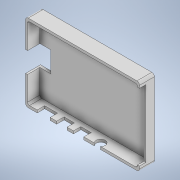
# Autodesk Inventor part: Pi 4 Case - Back Panel
Saved by Autodesk Inventor 2020 (Build 240168000, 168)
## iProperties
Created: 2021-01-01
Part Number: Pi 4 Case - Back Panel
Material: Generic
Document SubType Name: Modeling
Designer: frost
Density: 1 g/cm^3
Appearance: Default
Author: frost
Autodesk Inventor part; units mm, degrees
ref_plane "YZ Plane" through (0, 0, 0) normal (1, 0, 0) x (0, 1, 0)
ref_plane "XZ Plane" through (0, 0, 0) normal (0, 1, 0) x (-1, 0, 0)
ref_plane "XY Plane" through (0, 0, 0) normal (0, 0, 1) x (1, 0, 0)
sketch "Sketch1" plane through (0, 0, 0) normal (0, 0, 1) x (1, 0, 0)
  line L0 (-42, 30) -> (42, 30)
  line L1 (44, 28) -> (44, -28)
  line L2 (42, -30) -> (-42, -30)
  line L3 (-44, -28) -> (-44, 28)
  line L4 (-44, 30) -> (44, -30) construction
  line L5 (44, 30) -> (-44, -30) construction
  line L6 (-41.0667, 28) -> (41.0667, 28)
  line L7 (42.5, 26.5) -> (42.5, -26.5)
  line L8 (41.0667, -28) -> (-41.0667, -28)
  line L9 (-42.5, -26.5) -> (-42.5, 26.5)
  line L10 (-42.5, 28) -> (42.5, -28) construction
  line L11 (42.5, 28) -> (-42.5, -28) construction
  arc A0 (-41, 28) -> (-42.5, 26.5) centre (-41, 26.5) ccw
  arc A1 (42.5, 26.5) -> (41, 28) centre (41, 26.5) ccw
  arc A2 (41, -28) -> (42.5, -26.5) centre (41, -26.5) ccw
  arc A3 (-42.5, -26.5) -> (-41, -28) centre (-41, -26.5) ccw
  arc A4 (-44, -28) -> (-42, -30) centre (-42, -28) ccw
  arc A5 (-42, 30) -> (-44, 28) centre (-42, 28) ccw
  arc A6 (44, 28) -> (42, 30) centre (42, 28) ccw
  arc A7 (42, -30) -> (44, -28) centre (42, -28) ccw
  point P0 (0, 0)
  dimension "d0" = 88
  dimension "d1" = 60
  dimension "d2" = 85
  dimension "d3" = 56
  dimension "d4" = 3
  dimension "d5" = 3
  dimension "d6" = 2
  constraints: 24 end point, 16 point on circle, 16 point on line, 16 tangent, 8 centre point, 6 equal radius, 4 midpoint, 4 parallel, 2 horizontal, 2 perpendicular
  measures "d0" distance of L4.end L5.end
  measures "d1" distance of L5.start L4.end
  measures "d2" distance of L10.end L11.end
  measures "d3" distance of L11.start L10.end
  measures "d4" diameter of A3
  measures "d5" diameter of A2
  measures "d6" radius of A4
extrude "Extrusion1" add sketch "Sketch1" against normal blind 2 contours L0 A6 L1 A7 L2 A4 L3 A5 | L6 A1 L7 A2 L8 A3 L9 A0
extrude "Extrusion2" add sketch "Sketch1" along normal blind 9.5
sketch "Sketch2" plane through (44, -28, -2) normal (1, 0, 0) x (0, 0, -1)
  point P0 (-2, 28)
sketch "Sketch3" plane through (44, -28, -2) normal (1, 0, 0) x (0, 0, -1)
  line L0 (0, -2) -> (-11.5, -2) projected
  line L1 (-11.5, -2) -> (-11.5, 2)
  line L2 (-11.5, 1.5) -> (-11.5, 54.5) projected
  line L3 (-11.5, 2) -> (-6.5, 2)
  line L4 (-6.5, 2) -> (-6.5, 58)
  line L5 (0, 58) -> (-11.5, 58) projected
  line L6 (-11.5, 58) -> (-11.5, 54)
  line L7 (-11.5, 54) -> (-6.5, 54)
  line L8 (-11.5, 54) -> (-11.5, 2)
  point P0 (-2, 28)
  dimension "d11" = 4
  dimension "d12" = 5
  dimension "d13" = 4
  dimension "d14" = 53
  constraints: 12 end point, 4 perpendicular, 4 point on line
  measures "d11" distance of L0.end L1.end
  measures "d12" distance of L1.end L3.end
  measures "d13" distance of L5.end L6.end
  measures "d14" distance of L2.start L2.end
extrude "Extrusion3" cut sketch "Sketch3" against normal mid plane 9.5 contours L2 L7 L4 L3
sketch "Sketch4" plane through (-42, -30, -2) normal (0, -1, 0) x (1, 0, 0)
  line L0 (84, 0) -> (86, 0) projected
  circle A0 centre (53.5, 9) radius 3.5
  line L1 (18.9875, 0) -> (24.4875, 0)
  line L2 (-2, 0) -> (-2, 11.5) projected
  line L3 (43, 5.8) -> (43, 11.5)
  line L4 (35, 5.8) -> (35, 11.5)
  line L5 (30, 5.8) -> (30, 11.5)
  line L6 (22, 5.8) -> (22, 11.5)
  line L7 (17, 5.8) -> (17, 11.5)
  line L8 (7, 5.8) -> (7, 11.5)
  line L9 (83, 11.5) -> (1, 11.5) projected
  line L10 (17, 11.5) -> (7, 11.5)
  line L11 (22, 11.5) -> (30, 11.5)
  line L12 (35, 11.5) -> (43, 11.5)
  line L13 (86, 0) -> (86, 11.5) projected
  line L14 (84, 0) -> (0, 0) projected
  line L15 (7, 5.8) -> (17, 5.8)
  line L16 (22, 5.8) -> (30, 5.8)
  line L17 (35, 5.8) -> (43, 5.8)
  point P0 (42, 2)
  point P1 (55.9495, 11.5)
  point P2 (51.0505, 11.5)
  dimension "d19" = 7
  dimension "d22" = 8
  dimension "d23" = 5
  dimension "d24" = 8
  dimension "d25" = 5
  dimension "d26" = 10
  dimension "d27" = 32.5
  dimension "d28" = 9
  dimension "d29" = 5.8
  dimension "d38" = 10.5
  constraints: 26 end point, 6 point on line, 6 vertical, 3 horizontal, 1 centre point
  measures "d19" diameter of A0
  measures "d22" distance between parallel lines of L3 L4
  measures "d23" distance between parallel lines of L5 L4
  measures "d24" distance between parallel lines of L6 L5
  measures "d25" distance between parallel lines of L7 L6
  measures "d26" distance between parallel lines of L7 L8
  measures "d27" distance from line of L13 A0.centre
  measures "d28" distance from line of L14 A0.centre
  measures "d29" distance between parallel lines of L14 L15
  measures "d38" distance from line of L3 A0.centre
extrude "Extrusion4" cut sketch "Sketch4" against normal blind 9.5 contours A0 L9 | L7 L15 L8 L9 | L5 L16 L6 L9 | L3 L17 L4 L9 picked at (52.2452, 9.1659)
sketch "Sketch5" plane through (0, 0, -2) normal (0, 0, -1) x (-1, 0, 0)
  line L0 (44, -8) -> (34, -8)
  line L1 (34, -8) -> (34, 8)
  line L2 (34, 8) -> (44, 8)
  line L3 (44, 8) -> (44, -8)
  line L4 (-42, -30) -> (42, -30) projected
  line L5 (42, 30) -> (-42, 30) projected
  line L6 (44, -28) -> (44, 28) projected
  point P0 (0, 0)
  dimension "d32" = 22
  dimension "d33" = 22
  dimension "d34" = 0
  dimension "d35" = 10
  constraints: 8 end point, 2 parallel, 1 horizontal, 1 perpendicular
  measures "d32" distance between parallel lines of L4 L0
  measures "d33" distance between parallel lines of L5 L2
  measures "d34" distance between parallel lines of L6 L3
  measures "d35" distance of L0.start L0.end
extrude "Extrusion5" cut sketch "Sketch5" against normal blind 15
body "Solid1"
